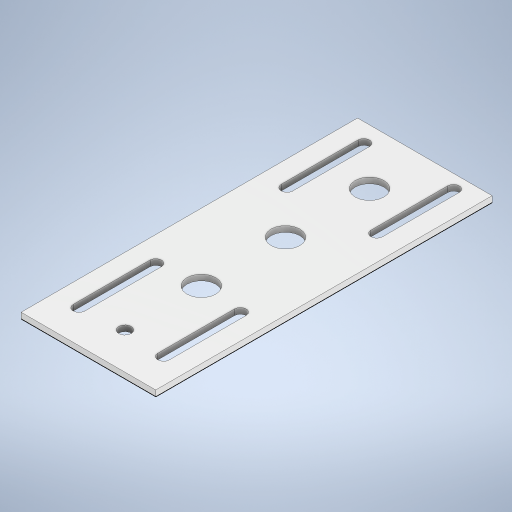
# Autodesk Inventor part: Sliding Plate
Saved by Autodesk Inventor 2023 (Build 270158000, 158)
## iProperties
Created: 2022-06-19
Part Number: Sliding Plate
Material: PVC, Unplasticized
Document SubType Name: Modeling
Designer: Shivan
Density: 1.29 g/cm^3
Appearance: Smooth - White
Author: Shivan
Autodesk Inventor part; units mm, degrees
ref_plane "YZ Plane" through (0, 0, 0) normal (1, 0, 0) x (0, 1, 0)
ref_plane "XZ Plane" through (0, 0, 0) normal (0, 1, 0) x (-1, 0, 0)
ref_plane "XY Plane" through (0, 0, 0) normal (0, 0, 1) x (1, 0, 0)
sketch "Sketch1" plane through (0, 0, 0) normal (0, 1, 0) x (-1, 0, 0)
  line L0 (0, 0) -> (70, 0)
  line L1 (70, 0) -> (70, -175)
  line L2 (70, -175) -> (0, -175)
  line L3 (0, -175) -> (0, 0)
  dimension "d0" = 70
  dimension "d1" = 175
  constraints: 8 end point, 2 parallel, 1 horizontal, 1 perpendicular
  measures "d0" distance of L1.end L2.end
  measures "d1" distance of L0.end L1.end
sketch "Sketch2" plane through (0, 0, 0) normal (0, 1, 0) x (-1, 0, 0)
  circle A0 centre (35, -58.75) radius 7.5
  circle A1 centre (35, -102.5) radius 7.5
  circle A2 centre (35, -146.25) radius 7.5
  line L0 (57, -17.0534) -> (57, -57.0534) construction
  line L1 (60, -17.0534) -> (60, -57.0534)
  line L2 (54, -57.0534) -> (54, -17.0534)
  arc A3 (60, -17.0534) -> (54, -17.0534) centre (57, -17.0534) ccw
  arc A4 (54, -57.0534) -> (60, -57.0534) centre (57, -57.0534) ccw
  line L3 (13, -17.0534) -> (13, -57.0534) construction
  line L4 (16, -17.0534) -> (16, -57.0534)
  line L5 (10, -57.0534) -> (10, -17.0534)
  arc A5 (16, -17.0534) -> (10, -17.0534) centre (13, -17.0534) ccw
  arc A6 (10, -57.0534) -> (16, -57.0534) centre (13, -57.0534) ccw
  line L6 (57, -125.2555) -> (57, -165.2555) construction
  line L7 (60, -125.2555) -> (60, -165.2555)
  line L8 (54, -165.2555) -> (54, -125.2555)
  arc A7 (60, -125.2555) -> (54, -125.2555) centre (57, -125.2555) ccw
  arc A8 (54, -165.2555) -> (60, -165.2555) centre (57, -165.2555) ccw
  line L9 (13, -127.9598) -> (13, -167.9598) construction
  line L10 (16, -127.9598) -> (16, -167.9598)
  line L11 (10, -167.9598) -> (10, -127.9598)
  arc A9 (16, -127.9598) -> (10, -127.9598) centre (13, -127.9598) ccw
  arc A10 (10, -167.9598) -> (16, -167.9598) centre (13, -167.9598) ccw
  line L12 (70, -175) -> (0, -175)
  line L13 (0, -175) -> (0, 0)
  line L14 (0, 0) -> (70, 0)
  line L15 (70, 0) -> (70, -175)
  point P0 (57, -37.0534)
  point P1 (13, -37.0534)
  point P2 (57, -145.2555)
  point P3 (13, -147.9598)
  point P4 (54, -37.0534)
  point P5 (60, -37.0534)
  point P6 (54, -145.2555)
  point P7 (60, -145.2555)
  point P8 (10, -147.9598)
  point P9 (16, -147.9598)
  point P10 (10, -37.0534)
  point P11 (16, -37.0534)
  point P12 (35, -175)
  dimension "d3" = 15
  dimension "d13" = 40
  dimension "d14" = 40
  dimension "d15" = 40
  dimension "d16" = 40
  dimension "d19" = 6
  dimension "d20" = 6
  dimension "d21" = 6
  dimension "d22" = 6
  dimension "d23" = 15
  dimension "d24" = 15
  dimension "d27" = 70
  dimension "d28" = 175
  dimension "d29" = 10
  dimension "d30" = 10
  dimension "d31" = 10
  dimension "d32" = 10
  dimension "d33" = 35
  dimension "d34" = 35
  dimension "d35" = 35
  dimension "d36" = 28.75
  dimension "d37" = 43.75
  dimension "d38" = 43.75
  constraints: 40 end point, 16 point on circle, 16 tangent, 13 midpoint, 11 centre point, 6 parallel, 4 vertical, 1 horizontal, 1 perpendicular
  measures "d3" diameter of A1
  measures "d13" distance of L6.start L6.end
  measures "d14" distance of L9.start L9.end
  measures "d15" distance of L0.start L0.end
  measures "d16" distance of L3.start L3.end
  measures "d19" distance of point (54, -37.053) point (60, -37.053)
  measures "d20" distance of point (54, -145.256) point (60, -145.256)
  measures "d21" distance of point (10, -147.96) point (16, -147.96)
  measures "d22" distance of point (10, -37.053) point (16, -37.053)
  measures "d23" diameter of A2
  measures "d24" diameter of A0
  measures "d27" distance of L12.start L12.end
  measures "d28" distance of L14.end L12.start
  measures "d29" distance from line of L15 point (60, -145.256)
  measures "d30" distance from line of L15 point (60, -37.053)
  measures "d31" distance from line of L13 point (10, -147.96)
  measures "d32" distance from line of L13 point (10, -37.053)
  measures "d33" distance from line of L15 A2.centre
  measures "d34" distance from line of L15 A1.centre
  measures "d35" distance from line of L15 A0.centre
  measures "d36" distance of point (35, -175) A2.centre
  measures "d37" distance of A1.centre A2.centre
  measures "d38" distance of A1.centre A0.centre
extrude "Extrusion1" add sketch "Sketch1" along normal blind 3
extrude "Extrusion2" cut sketch "Sketch2" along normal blind 10 contours A0 | A1 | A2 | L1 A4 L2 A3 | L4 A6 L5 A5 | L7 A8 L8 A7 | L10 A10 L11 A9
sketch "Sketch6" plane through (0, 3, 0) normal (0, 1, 0) x (1, 0, 0)
  arc A0 (-38.25, 19) -> (-31.75, 19) centre (-35, 19) ccw
  arc A1 (-31.75, 19) -> (-38.25, 19) centre (-35, 19) ccw
  line L0 (0, 175) -> (-70, 175) projected
  line L1 (0, 0) -> (0, 175) projected
  line L2 (-70, 175) -> (0, 175)
  line L3 (0, 175) -> (0, 0)
  line L4 (0, 0) -> (-70, 0)
  line L5 (-70, 0) -> (-70, 175)
  line L6 (-70, 0) -> (0, 0) projected
  point P0 (-35, 19)
  point P1 (-31.75, 19)
  point P2 (-35, 0)
  point P3 (-35, 0)
  point P4 (-35, 15.75)
  dimension "d9" = 0
  dimension "d39" = 6.5
  dimension "d40" = 35
  dimension "d41" = 19
  dimension "d42" = 15.75
  constraints: 8 end point, 5 point on circle, 2 centre point, 2 midpoint, 2 parallel, 1 coincident, 1 horizontal, 1 perpendicular, 17 other
  measures "d9" distance of A0.centre A1.centre
  measures "d39" distance of point (-31.75, 19) point (-38.25, 19)
  measures "d40" distance from line of L5 A0.centre
  measures "d41" distance of point (-35, 0) A0.centre
  measures "d42" distance of point (-35, 0) point (-35, 15.75)
extrude "Extrusion3" cut sketch "Sketch6" against normal blind 10 contours A1 A0
body "Solid1"
